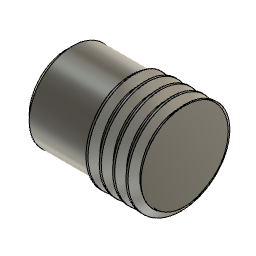
thread18M (Autodesk Fusion 360 design; units mm, degrees)
Autodesk Fusion 360 part; units mm, degrees
sketch "Sketch1" plane through (0, 0, 0) normal (1, 0, 0) x (0, 1, 0)
  circle A0 centre (0, 0) radius 8.1
  dimension "d1" = 16.2
  constraint coincident A0.centre origin
  measures "d1" diameter of A0
extrude "Extrude1" add sketch "Sketch1" against normal blind 12
sketch "Sketch2" plane through (0, 0, 0) normal (1, 0, 0) x (0, 1, 0)
  circle A0 centre (0, 0) radius 8.1
  circle A1 centre (0, 0) radius 9
  dimension "d4" = 18
  constraint coincident A0.centre A1.centre
  measures "d4" diameter of A1
extrude "Extrude2" add sketch "Sketch2" along normal blind 10 contours A0 | A1
thread "Thread1" "ISO Metric profile 18.0 M18x2.5 4g6g" major diameter 17.7905 minor diameter 14.9699 pitch 2.5 angle 60 modelled right hand crest width 0.3786 on face at (6.6667, 8.9888, -0.4486) crest through (-0.625, 8.8953, 0)
chamfer "Chamfer1" distance 1 angle 45 1 edges at (-12, -7.5519, 2.9291)
